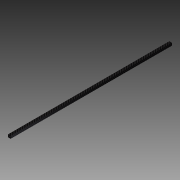
# Autodesk Inventor part: carbon_stick_gimbal
Saved by Autodesk Inventor 2015 SP1 (Build 190203100, 203)
## iProperties
Created: 2015-07-15
Part Number: carbon_stick_gimbal
Material: Generic
Document SubType Name: Modeling
Designer: Alexandre Cherpillod
Density: 1 g/cm^3
Appearance: Carbon Fiber
Author: Alexandre Cherpillod
Autodesk Inventor part; units mm, degrees
ref_plane "YZ Plane" through (0, 0, 0) normal (1, 0, 0) x (0, 1, 0)
ref_plane "XZ Plane" through (0, 0, 0) normal (0, 1, 0) x (-1, 0, 0)
ref_plane "XY Plane" through (0, 0, 0) normal (0, 0, 1) x (1, 0, 0)
sketch "Sketch1" plane through (0, 0, 0) normal (0, 1, 0) x (-1, 0, 0)
  line L0 (0, 0) -> (4, 0)
  line L1 (4, 0) -> (4, -4)
  line L2 (4, -4) -> (0, -4)
  line L3 (0, -4) -> (0, 0)
  line L4 (3.25, -0.75) -> (0.75, -0.75)
  line L5 (0.75, -0.75) -> (0.75, -3.25)
  line L6 (0.75, -3.25) -> (3.25, -3.25)
  line L7 (3.25, -3.25) -> (3.25, -0.75)
  dimension "d0" = 4
  dimension "d1" = 4
  dimension "d4" = 0.75
  constraints: 16 end point, 4 parallel, 2 perpendicular, 1 horizontal, 3 other
  measures "d0" distance of L1.end L2.end
  measures "d1" distance of L0.end L1.end
  measures "d4" distance between parallel lines of L0 L4
extrude "Extrusion2" add sketch "Sketch1" along normal mid plane 250
body "Solid2"
